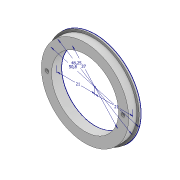
# Autodesk Inventor part: Adapter-D37mm-SM2
Saved by Autodesk Inventor 2021 (Build 250183000, 183)
## iProperties
Created: 2022-09-26
Part Number: Adapter-D37mm-SM2
Material: Generic
Document SubType Name: Modeling
Designer: nvladi
Density: 1 g/cm^3
Appearance: Default
Author: nvladi
Autodesk Inventor part; units mm, degrees
ref_plane "YZ Plane" through (0, 0, 0) normal (1, 0, 0) x (0, 1, 0)
ref_plane "XZ Plane" through (0, 0, 0) normal (0, 1, 0) x (-1, 0, 0)
ref_plane "XY Plane" through (0, 0, 0) normal (0, 0, 1) x (1, 0, 0)
sketch "Sketch1" plane through (0, 0, 0) normal (0, 0, 1) x (1, 0, 0)
  circle A0 centre (0, 0) radius 18.5
  circle A1 centre (0, 0) radius 24.125
  circle A2 centre (0, 0) radius 25.4
  point P0 (-21, 0)
  point P1 (21, 0)
  dimension "d0" = 37
  dimension "d1" = 48.25
  dimension "d2" = 50.8
  dimension "d14" = 21
  dimension "d15" = 21
  constraints: 3 centre point, 3 coincident
  measures "d0" diameter of A0
  measures "d1" diameter of A1
  measures "d2" diameter of A2
  measures "d14" distance of point (0, 0) point (-21, 0)
  measures "d15" distance of point (21, 0) point (0, 0)
extrude "Extrusion1" add sketch "Sketch1" along normal blind 5.5 contours A1
extrude "Extrusion2" add sketch "Sketch1" along normal blind 1 contours A2
hole "Hole1" at (-21, 0, 0) at (21, 0, 0) direction (0, 0, 1) diameter 2 end through all
body "Solid1"
